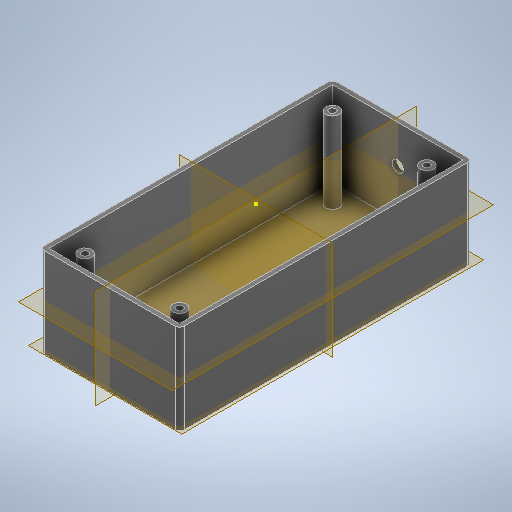
# Autodesk Inventor part: Resistencia_Cuerpo
Saved by Autodesk Inventor 2026 (Build 300175050, 175E)
## iProperties
Created: 2025-05-26
Part Number: Resistencia_Cuerpo
Material: PVC, no plastificado
Document SubType Name: Modeling
Designer: alex
Density: 1.29 g/cm^3
Appearance: Suave - Blanco
Author: alex
Autodesk Inventor part; units mm, degrees
sketch "Cuerpo" plane through (0, 0, 0) normal (0, 1, 0) x (-1, 0, 0)
  line L0 (0, -91.5799) -> (0, 91.5799) projected
  line L1 (-43.9799, 0) -> (43.9799, 0) projected
  line L2 (29, -65) -> (-29, -65)
  line L3 (-31, -63) -> (-31, 63)
  line L4 (-29, 65) -> (29, 65)
  line L5 (31, 63) -> (31, -63)
  arc A0 (29, -65) -> (31, -63) centre (29, -63) ccw
  arc A1 (-31, -63) -> (-29, -65) centre (-29, -63) ccw
  arc A2 (31, 63) -> (29, 65) centre (29, 63) ccw
  arc A3 (-29, 65) -> (-31, 63) centre (-29, 63) ccw
  circle A4 centre (21, -55) radius 1.5
  circle A5 centre (21, -55) radius 3
  circle A6 centre (-21, -55) radius 1.5
  circle A7 centre (-21, -55) radius 3
  circle A8 centre (21, 55) radius 1.5
  circle A9 centre (21, 55) radius 3
  circle A10 centre (-21, 55) radius 3
  circle A11 centre (-21, 55) radius 1.5
  line L6 (29, -63) -> (-29, -63)
  line L7 (-29, -63) -> (-29, 63)
  line L8 (-29, 63) -> (29, 63)
  line L9 (29, 63) -> (29, -63)
  point P0 (0, 0)
  point P1 (31, -65)
  point P2 (-31, 65)
  dimension "d0" = 31
  dimension "d1" = 65
  dimension "d2" = 31
  dimension "d3" = 65
  dimension "d4" = 2
  dimension "d5" = 10
  dimension "d6" = 10
  dimension "d7" = 10
  dimension "d8" = 10
  dimension "d9" = 10
  dimension "d10" = 10
  dimension "d11" = 10
  dimension "d12" = 10
  dimension "d13" = 3
  dimension "d14" = 6
  dimension "d15" = 3
  dimension "d16" = 6
  dimension "d17" = 3
  dimension "d18" = 6
  dimension "d19" = 6
  dimension "d20" = 3
  constraints: 16 end point, 12 centre point, 8 coincident, 8 point on circle, 8 tangent, 4 parallel, 4 point on line, 3 equal radius, 2 horizontal, 2 perpendicular
  measures "d0" distance from line of L0 point (31, -65)
  measures "d1" distance from line of L1 point (31, -65)
  measures "d2" distance from line of L0 point (-31, 65)
  measures "d3" distance from line of L1 point (-31, 65)
  measures "d4" radius of A0
  measures "d5" distance from line of L5 point (21, -55)
  measures "d6" distance from line of L2 point (21, -55)
  measures "d7" distance from line of L2 point (-21, -55)
  measures "d8" distance from line of L3 point (-21, -55)
  measures "d9" distance from line of L5 point (21, 55)
  measures "d10" distance from line of L4 point (21, 55)
  measures "d11" distance from line of L4 point (-21, 55)
  measures "d12" distance from line of L3 point (-21, 55)
  measures "d13" diameter of A4
  measures "d14" diameter of A5
  measures "d15" diameter of A6
  measures "d16" diameter of A7
  measures "d17" diameter of A8
  measures "d18" diameter of A9
  measures "d19" diameter of A10
  measures "d20" diameter of A11
extrude "Extrusión1" add sketch "Cuerpo" along normal mid plane 38 contours L2 A1 L3 L1 L7 L6 L0 | L0 L6 L9 L1 L5 A0 L2 | L8 L7 L1 L3 A3 L4 L0 | L0 L4 A2 L5 L1 L9 L8 | A5 | A7 | A9 | A10
ref_plane "Plano de trabajo1" through (0, -19, 0) normal (0, 1, 0) x (-1, 0, 0)
sketch "Boceto2" plane through (0, -19, 0) normal (0, 1, 0) x (-1, 0, 0)
  line L0 (-29, -65) -> (29, -65)
  line L1 (31, -63) -> (31, 63)
  line L2 (29, 65) -> (-29, 65)
  line L3 (-31, 63) -> (-31, -63)
  arc A0 (-31, -63) -> (-29, -65) centre (-29, -63) ccw
  arc A1 (29, -65) -> (31, -63) centre (29, -63) ccw
  arc A2 (-29, 65) -> (-31, 63) centre (-29, 63) ccw
  arc A3 (31, 63) -> (29, 65) centre (29, 63) ccw
  line L4 (-43.9799, 0) -> (43.9799, 0) projected
  line L5 (0, -91) -> (0, 91) projected
  point P0 (0, 0)
  dimension "d24" = 2
  dimension "d34" = 65
  dimension "d35" = 65
  dimension "d36" = 31
  constraints: 8 end point, 8 point on circle, 8 tangent, 4 centre point, 3 equal radius, 2 parallel, 1 horizontal, 1 perpendicular
  measures "d24" radius of A0
  measures "d34" distance between parallel lines of L4 L2
  measures "d35" distance between parallel lines of L4 L0
  measures "d36" distance between parallel lines of L5 L1
extrude "Base" add sketch "Boceto2" against normal blind 2
sketch "Boceto3" plane through (29, 19, -65) normal (0, 0, -1) x (-1, 0, 0)
  line L0 (58, -40) -> (0, -40) projected
  line L1 (-2, -40) -> (-2, 0) projected
  circle A0 centre (29, -17) radius 2.5
  point P0 (29, -19)
  dimension "d27" = 23
  dimension "d28" = 31
  dimension "d29" = 5
  constraints: 1 centre point, 1 coincident
  measures "d27" distance from line of L0 point (29, -17)
  measures "d28" distance from line of L1 point (29, -17)
  measures "d29" diameter of A0
extrude "Extrusión3" cut sketch "Boceto3" against normal blind 125
sketch "Boceto4" plane through (-21, 19, 55) normal (0, 1, 0) x (1, 0, 0)
  point P0 (21, 55)
sketch "Boceto5" plane through (-21, 19, 55) normal (0, 1, 0) x (1, 0, 0)
  circle A0 centre (0, 0) radius 1.5 projected
  circle A1 centre (0, 0) radius 3
  circle A2 centre (0, 110) radius 1.5 projected
  circle A3 centre (0, 110) radius 3
  circle A4 centre (42, 110) radius 1.5 projected
  circle A5 centre (42, 110) radius 3
  circle A6 centre (42, 0) radius 1.5 projected
  circle A7 centre (42, 0) radius 3
  point P0 (21, 55)
  constraints: 4 centre point, 4 coincident
extrude "Extrusión4" cut sketch "Boceto5" against normal blind 2 contours A1 | A2 | A3 | A4 | A5 | A7
equation "\"d2\" = d0"
equation "\"d3\" = d1"
equation "\"d6\" = d5"
equation "\"d7\" = d5"
equation "\"d8\" = d5"
equation "\"d9\" = d5"
equation "\"d10\" = d5"
equation "\"d11\" = d5"
equation "\"d12\" = d5"
equation "\"d15\" = d13"
equation "\"d16\" = d14"
equation "\"d17\" = d13"
equation "\"d18\" = d14"
equation "\"d19\" = d14"
equation "\"d20\" = d13"
